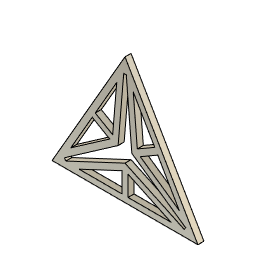
零件2 v3 (Autodesk Fusion 360 design; units mm, degrees)
Autodesk Fusion 360 part; units mm, degrees
sketch "草图1" plane through (0, 0, 0) normal (0, 1, 0) x (1, 0, 0)
  line L0 (2.4024, -17.839) -> (16.6502, 6.839)
  line L1 (-16.6502, 6.839) -> (-2.4024, -17.839)
  arc A0 (-14.2478, 11) -> (-16.6502, 6.839) centre (0, 0) ccw
  line L2 (14.2478, 11) -> (-14.2478, 11)
  arc A1 (16.6502, 6.839) -> (14.2478, 11) centre (0, 0) ccw
  arc A2 (-2.4024, -17.839) -> (2.4024, -17.839) centre (0, 0) ccw
  line L3 (12.1244, 7) -> (-12.1244, 7)
  line L4 (-12.1244, 7) -> (0, -14)
  line L5 (0, -14) -> (12.1244, 7)
  line L6 (0, -14) -> (1.1374, -0.6567)
  line L7 (12.1244, 7) -> (1.1374, -0.6567)
  line L8 (1.3775, -9.6141) -> (2.0939, -1.2089)
  line L9 (9.0148, 3.6141) -> (2.0939, -1.2089)
  line L10 (2.047, -1.7592) -> (4.9462, -3.433)
  line L11 (2.547, -0.8932) -> (5.4462, -2.567)
  line L12 (1.3775, -9.6141) -> (4.9462, -3.433)
  line L13 (5.4462, -2.567) -> (9.0148, 3.6141)
  line L14 (12.1244, 7) -> (0, 1.3134)
  line L15 (7.6373, 6) -> (0, 2.4179)
  line L16 (0.5, 2.6524) -> (0.5, 6)
  line L17 (-0.5, 2.6524) -> (-0.5, 6)
  line L18 (-7.6373, 6) -> (0, 2.4179)
  line L19 (-12.1244, 7) -> (0, 1.3134)
  line L20 (-0.5, 6) -> (-7.6373, 6)
  line L21 (7.6373, 6) -> (0.5, 6)
  line L22 (-12.1244, 7) -> (-1.1374, -0.6567)
  line L23 (-9.0148, 3.6141) -> (-2.0939, -1.2089)
  line L24 (-2.547, -0.8932) -> (-5.4462, -2.567)
  line L25 (-2.047, -1.7592) -> (-4.9462, -3.433)
  line L26 (-1.3775, -9.6141) -> (-2.0939, -1.2089)
  line L27 (0, -14) -> (-1.1374, -0.6567)
  line L28 (-4.9462, -3.433) -> (-1.3775, -9.6141)
  line L29 (-9.0148, 3.6141) -> (-5.4462, -2.567)
  circle A3 centre (0, -14) radius 2.5
  circle A4 centre (12.1244, 7) radius 2.5
  circle A5 centre (-12.1244, 7) radius 2.5
  dimension "d1" = -4
  dimension "d6" = 360
  dimension "d7" = 5
  dimension "d9" = 360
  constraint coincident A0.centre A1.centre
  constraint coincident L8 L10.start
  constraint coincident L11.end L12
  constraint collinear L12 L13
  constraint coincident L9 L11.start
  constraint coincident L4.end L5.start
  measures "d7" diameter of A3
extrude "拉伸1" add sketch "草图1" along normal blind 1 contours L3 L19 A5 | L3 L14 L19 A4 A5 | L4 L22 A5 | L19 L22 A5 | L3 L14 A4 | L4 L22 L27 A3 A5 | L5 L7 A4 | L7 L14 A4 | L4 L27 A3 | L5 L6 L7 A3 A4 | L5 L6 A3 | L6 L27 A3
